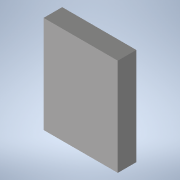
# Autodesk Inventor part: Foam_Front
Saved by Autodesk Inventor 2021 (Build 250183000, 183)
## iProperties
Created: 2021-02-18
Part Number: Foam_Front
Material: Polystyrene, Expanded
Document SubType Name: Modeling
Designer: negt20
Density: 0.05 g/cm^3
Appearance: Gray
Author: negt20
Autodesk Inventor part; units mm, degrees
ref_plane "YZ Plane" through (0, 0, 0) normal (1, 0, 0) x (0, 1, 0)
ref_plane "XZ Plane" through (0, 0, 0) normal (0, 1, 0) x (-1, 0, 0)
ref_plane "XY Plane" through (0, 0, 0) normal (0, 0, 1) x (1, 0, 0)
sketch "Sketch1" plane through (0, 0, 0) normal (0, 0, 1) x (1, 0, 0)
  line L0 (-50, 65.5) -> (50, 65.5)
  line L1 (50, 65.5) -> (50, -65.5)
  line L2 (50, -65.5) -> (-50, -65.5)
  line L3 (-50, -65.5) -> (-50, 65.5)
  point P0 (0, 0)
  point P1 (0, 65.5)
  point P2 (-50, 0)
  dimension "d0" = 100
  dimension "d1" = 131
  constraints: 8 end point, 2 midpoint, 2 parallel, 1 horizontal, 1 horizontal alignment, 1 perpendicular, 1 vertical alignment
  measures "d0" distance of L1.end L2.end
  measures "d1" distance of L0.end L1.end
extrude "Extrusion1" add sketch "Sketch1" along normal blind 25
body "Solid1"
